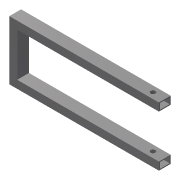
# Autodesk Inventor part: GARFO
Saved by Autodesk Inventor 2015 (Build 190159000, 159)
## iProperties
Created: 2016-08-09
Part Number: GARFO
Material: Aluminium AW-7020
Document SubType Name: Modeling
Designer: EriveltonDell
Density: 2.78 g/cm^3
Appearance: Stainless - Brushed
Mass: 1234.07 g
Surface Area: 731.335 cm^2
Volume: 443.911 cm^3
Author: EriveltonDell
Autodesk Inventor part; units mm, degrees
ref_plane "YZ Plane" through (0, 0, 0) normal (1, 0, 0) x (0, 1, 0)
ref_plane "XZ Plane" through (0, 0, 0) normal (0, 1, 0) x (-1, 0, 0)
ref_plane "XY Plane" through (0, 0, 0) normal (0, 0, 1) x (1, 0, 0)
sketch "Sketch1" plane through (0, 0, 0) normal (0, 1, 0) x (-1, 0, 0)
  line L0 (0, 0) -> (370, 0)
  line L1 (370, 0) -> (370, 130)
  line L2 (370, 130) -> (0, 130)
  dimension "d7" = 370
  dimension "d8" = 130
  dimension "d9" = 370
  constraints: 10 end point, 2 perpendicular, 1 horizontal
  measures "d7" distance of L0.start L0.end
  measures "d8" distance of L0.end L1.end
  measures "d9" distance of L1.end L2.end
sketch "Sketch2" plane through (0, 0, 0) normal (1, 0, 0) x (0, 1, 0)
  line L0 (0, 0) -> (-30, 0)
  line L1 (0, 0) -> (-15, 0)
  line L2 (-15, 0) -> (-15, -10)
  line L3 (-15, -10) -> (15, -10)
  line L4 (15, -10) -> (15, 10)
  line L5 (15, 10) -> (-15, 10)
  line L6 (-15, 10) -> (-15, 0)
  line L7 (12, 7) -> (12, -7)
  line L8 (12, -7) -> (-12, -7)
  line L9 (-12, -7) -> (-12, 0)
  line L10 (-12, 0) -> (-12, 7)
  line L11 (-12, 7) -> (12, 7)
  dimension "d20" = 15
  dimension "d21" = 10
  dimension "d22" = 30
  dimension "d23" = 20
  dimension "d24" = 30
  dimension "d25" = 3
  constraints: 24 end point, 5 perpendicular, 2 collinear, 1 coincident, 1 horizontal, 1 midpoint, 1 point on line, 4 other
  measures "d20" distance of L0.start L1.end
  measures "d21" distance of L1.end L2.end
  measures "d22" distance of L2.end L3.end
  measures "d23" distance of L3.end L4.end
  measures "d24" distance of L4.end L5.end
  measures "d25" distance between parallel lines of L4 L7
sweep "Sweep1" add profiles "Sketch2" path "Sketch1" contours L6 L5 L4 L3 L2 | L7 L8 L9 L10 L11
sketch "Sketch3" plane through (0, 0, 0) normal (0, 0, 1) x (1, 0, 0)
  line L0 (0, 0) -> (-30, 0)
  circle A0 centre (-30, 0) radius 6
  dimension "d14" = 30
  dimension "d15" = 12
  constraints: 2 end point, 1 centre point, 1 coincident, 1 horizontal
  measures "d14" distance of L0.start L0.end
  measures "d15" diameter of A0
extrude "Extrusion1" cut sketch "Sketch3" along normal through all both and the other way through all
shell "Shell1" thickness 2.5 removed faces 1 at (0, -5, 133.3333)
shell "Shell2" thickness 2.5 removed faces 3 at (0, -5, -3.3333) at (0, -4.1667, 120.8333) at (-2.5, -4.1667, -2.5)
body "Solid1"
